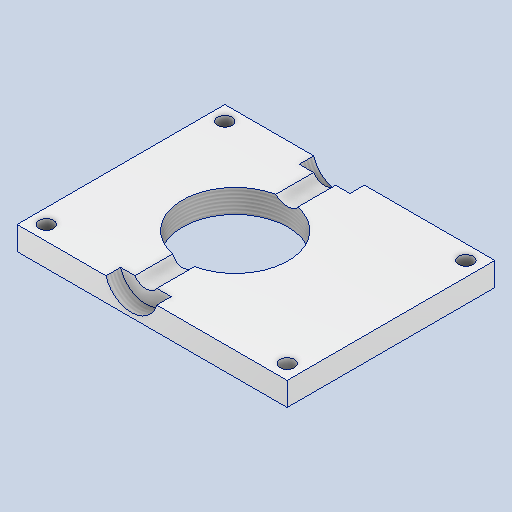
# Autodesk Inventor part: CuvetteHolderFace
Saved by Autodesk Inventor 2022 (Build 260153000, 153)
## iProperties
Created: 2021-04-01
Part Number: CuvetteHolderFace
Material: Aluminum 6061
Document SubType Name: Modeling
Designer: wilso
Density: 2.7 g/cm^3
Appearance: Aluminum - Flat
Author: wilso
Autodesk Inventor part; units mm, degrees
ref_plane "YZ Plane" through (0, 0, 0) normal (1, 0, 0) x (0, 1, 0)
ref_plane "XZ Plane" through (0, 0, 0) normal (0, 1, 0) x (-1, 0, 0)
ref_plane "XY Plane" through (0, 0, 0) normal (0, 0, 1) x (1, 0, 0)
sketch "Sketch1" plane through (0, 0, 0) normal (0, 1, 0) x (-1, 0, 0)
  line L0 (0, 0) -> (65, 0)
  line L1 (65, 0) -> (65, -50)
  line L2 (65, -50) -> (0, -50)
  line L3 (0, -50) -> (0, 0)
  circle A0 centre (37.5, -25) radius 12.7
  dimension "d0" = 65
  dimension "d1" = 50
  dimension "d2" = 25.4
  dimension "d3" = 27.5
  constraints: 8 end point, 2 parallel, 1 centre point, 1 horizontal, 1 perpendicular
  measures "d0" distance of L1.end L2.end
  measures "d1" distance of L0.end L1.end
  measures "d2" diameter of A0
  measures "d3" distance from line of L1 A0.centre
extrude "Extrusion1" add sketch "Sketch1" along normal blind 5.65
thread "Thread1" size "1-32 UN" class "2B" standard "ANSI Unified Screw Threads" full length
sketch "Sketch2" plane through (0, 5.65, 0) normal (0, 1, 0) x (1, 0, 0)
  line L0 (-65, 0) -> (0, 0) projected
  line L1 (-65, 50) -> (-65, 0) projected
  line L2 (0, 0) -> (0, 50) projected
  line L3 (0, 50) -> (-65, 50) projected
  point P0 (-61.5, 3.5)
  point P1 (-3.5, 3.5)
  point P2 (-3.5, 46.5)
  point P3 (-61.5, 46.5)
  dimension "d15" = 3.5
  dimension "d16" = 3.5
  dimension "d17" = 3.5
  dimension "d18" = 3.5
  dimension "d19" = 3.5
  dimension "d20" = 3.5
  dimension "d21" = 3.5
  dimension "d22" = 3.5
  measures "d15" distance from line of L0 point (-61.5, 3.5)
  measures "d16" distance from line of L1 point (-61.5, 3.5)
  measures "d17" distance from line of L0 point (-3.5, 3.5)
  measures "d18" distance from line of L2 point (-3.5, 3.5)
  measures "d19" distance from line of L2 point (-3.5, 46.5)
  measures "d20" distance from line of L3 point (-3.5, 46.5)
  measures "d21" distance from line of L3 point (-61.5, 46.5)
  measures "d22" distance from line of L1 point (-61.5, 46.5)
hole "Hole1" at (-61.5, 5.65, -3.5) at (-3.5, 5.65, -3.5) at (-3.5, 5.65, -46.5) at (-61.5, 5.65, -46.5) direction (0, -1, 0) diameter 3.5 end through all
sketch "Sketch3" plane through (-65, 0, 0) normal (0, 0, 1) x (1, 0, 0)
  line L0 (14.8, 5.65) -> (40.2, 5.65) projected
  line L1 (27.5, 5.65) -> (27.5, 7.4)
  circle A0 centre (27.5, 7.4) radius 3.175
  circle A1 centre (27.5, 7.4) radius 6.35
  point P0 (65, 0)
  point P1 (21.3959, 5.65)
  point P2 (33.6041, 5.65)
  point P3 (30.1492, 5.65)
  point P4 (24.8508, 5.65)
  dimension "d23" = 1.75
  dimension "d24" = 6.35
  dimension "d25" = 12.7
  constraints: 2 centre point, 2 coincident, 2 end point, 1 midpoint, 1 vertical
  measures "d23" distance of L1.start L1.end
  measures "d24" diameter of A0
  measures "d25" diameter of A1
extrude "Extrusion2" cut sketch "Sketch3" against normal blind 60 contours A0 L0 | L0 A0
extrude "Extrusion3" cut sketch "Sketch3" against normal blind 3.5 contours L0 A0 A1 picked at (22.7391, 5.1926)
sketch "Sketch4" plane through (0, 0, -50) normal (0, 0, -1) x (-1, 0, 0)
  arc A0 (34.8508, 5.65) -> (40.1492, 5.65) centre (37.5, 7.4) ccw projected
  circle A1 centre (37.5, 7.4) radius 6.35
  point P0 (0, 0)
  dimension "d30" = 12.7
  constraints: 1 centre point, 1 coincident
  measures "d30" diameter of A1
extrude "Extrusion4" cut sketch "Sketch4" against normal blind 3.5
thread "Thread2" size "1/2-32 UN" class "2B" standard "ANSI Unified Screw Threads" full length
equation "\"d30\" = d25"
body "Solid1"
